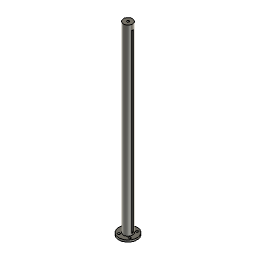
_Motorised arm.b936b334-40dd-4a6a-bc5e-916818be2f43 (Autodesk Fusion 360 design; units mm, degrees)
Autodesk Fusion 360 part; units mm, degrees
sketch "Sketch1" plane through (0, 0, 0) normal (0, 0, 1) x (1, 0, 0)
  circle A0 centre (0, 0) radius 25
  dimension "d1" = 50
  constraint coincident A0.centre origin
  measures "d1" diameter of A0
extrude "Extrude1" add sketch "Sketch1" along normal blind 5
sketch "Sketch2" plane through (0, 0, 5) normal (0, 0, 1) x (-1, 0, 0)
  circle A0 centre (0, 0) radius 25
  circle A1 centre (0, 0) radius 12.5
  dimension "d4" = 25
  constraint coincident A0.centre A1.centre
  measures "d4" diameter of A1
extrude "Extrude2" add sketch "Sketch2" along normal blind 500 contours A1
sketch "Sketch3" plane through (0, 0, 5) normal (0, 0, 1) x (-1, 0, 0)
  circle A0 centre (0, 0) radius 12.5
  circle A1 centre (0, 0) radius 25
  circle A2 centre (15, -10) radius 3
  circle A3 centre (-10, -15) radius 3
  circle A4 centre (-15, 10) radius 3
  circle A5 centre (10, 15) radius 3
  dimension "d7" = 6
  dimension "d8" = 6
  dimension "d9" = 6
  dimension "d10" = 6
  measures "d7" diameter of A2
  measures "d8" diameter of A3
  measures "d9" diameter of A4
  measures "d10" diameter of A5
extrude "Extrude3" cut sketch "Sketch3" against normal blind 5 contours A2 | A3 | A4 | A5
move_body "Move1" bodies 1 to x (1, 0, 0) y (0, 1, 0) z (0, 0, 1) at (-50, 0, 0)
sketch "Sketch4" plane through (0, 0, 0) normal (1, 0, 0) x (0, 1, 0)
  line L0 (-2, 10) -> (2, 10)
  line L1 (2, 10) -> (2, 490)
  line L2 (2, 490) -> (-2, 490)
  line L3 (-2, 490) -> (-2, 10)
  dimension "d13" = 4
  dimension "d14" = 480
  constraint horizontal L0
  constraint vertical L1
  constraint horizontal L2
  constraint vertical L3
  measures "d13" distance of L0.start L0.end
  measures "d14" distance of L0.start L2.end
extrude "Extrude4" cut sketch "Sketch4" against normal blind 100
sketch "Sketch5" plane through (0, 0, 505) normal (0, 0, 1) x (-1, 0, 0)
  circle A0 centre (50, 0) radius 12.5
  circle A1 centre (50, 0) radius 3
  dimension "d17" = 6
  constraint concentric A0 A1
  measures "d17" diameter of A1
extrude "Extrude5" cut sketch "Sketch5" against normal blind 5 contours A1
